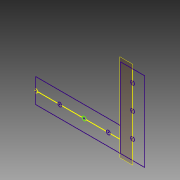
# Autodesk Inventor part: Bumper Holder
Saved by Autodesk Inventor 2014 (Build 180170000, 170)
## iProperties
Created: 2014-01-19
Part Number: Bumper Holder
Material: Generic
Document SubType Name: Sheet Metal
Designer: intern
Density: 1 g/cm^3
Sheet Metal Rule: Default
Appearance: Default
Author: intern
Autodesk Inventor part; units mm, degrees
ref_plane "YZ Plane" through (0, 0, 0) normal (1, 0, 0) x (0, 1, 0)
ref_plane "XZ Plane" through (0, 0, 0) normal (0, 1, 0) x (-1, 0, 0)
ref_plane "XY Plane" through (0, 0, 0) normal (0, 0, 1) x (1, 0, 0)
ref_plane "Work Plane1" through (7.5537, -38.3367, 0) normal (0, 0, 1) x (1, 0, 0)
sketch "Sketch1" plane through (7.5537, -38.3367, 0) normal (0, 0, 1) x (1, 0, 0)
  line L0 (-7.5537, -44.8483) -> (5.0701, -44.8483)
  line L1 (5.0701, -44.8483) -> (5.0701, -27.232)
  arc A0 (5.0701, -23.0946) -> (5.0701, -27.232) centre (5.1463, -25.1633) ccw
  line L2 (5.0701, -23.0946) -> (5.0701, -1.832)
  arc A1 (5.0701, 2.3054) -> (5.0701, -1.832) centre (5.1463, 0.2367) ccw
  line L3 (5.0701, 2.3054) -> (5.0701, 23.568)
  arc A2 (5.0701, 27.7054) -> (5.0701, 23.568) centre (5.1463, 25.6367) ccw
  line L4 (5.0701, 27.7054) -> (5.0701, 38.3367)
  line L5 (-7.5537, 38.3367) -> (5.0701, 38.3367)
  line L6 (-7.5537, 38.3367) -> (-7.5537, -44.8483)
  line L7 (5.2225, -44.8483) -> (17.8463, -44.8483)
  line L8 (17.8463, 38.3367) -> (17.8463, -44.8483)
  line L9 (5.2225, 38.3367) -> (17.8463, 38.3367)
  line L10 (5.2225, 27.7054) -> (5.2225, 38.3367)
  arc A3 (5.2225, 23.568) -> (5.2225, 27.7054) centre (5.1463, 25.6367) ccw
  line L11 (5.2225, 2.3054) -> (5.2225, 23.568)
  arc A4 (5.2225, -1.832) -> (5.2225, 2.3054) centre (5.1463, 0.2367) ccw
  line L12 (5.2225, -23.0946) -> (5.2225, -1.832)
  arc A5 (5.2225, -27.232) -> (5.2225, -23.0946) centre (5.1463, -25.1633) ccw
  line L13 (5.2225, -44.8483) -> (5.2225, -27.232)
  line L14 (-96.4537, -34.2184) -> (-96.4537, -44.8483)
  line L15 (-7.5537, -44.8483) -> (-96.4537, -44.8483)
  line L16 (-7.5537, -32.2245) -> (-7.5537, -44.8483)
  line L17 (-18.185, -32.2245) -> (-7.5537, -32.2245)
  arc A6 (-22.3224, -32.2245) -> (-18.185, -32.2245) centre (-20.2537, -32.1483) ccw
  line L18 (-43.585, -32.2245) -> (-22.3224, -32.2245)
  arc A7 (-47.7224, -32.2245) -> (-43.585, -32.2245) centre (-45.6537, -32.1483) ccw
  line L19 (-68.985, -32.2245) -> (-47.7224, -32.2245)
  arc A8 (-73.1224, -32.2245) -> (-68.985, -32.2245) centre (-71.0537, -32.1483) ccw
  line L20 (-94.385, -32.2245) -> (-73.1224, -32.2245)
  arc A9 (-96.4537, -34.2184) -> (-94.385, -32.2245) centre (-96.4537, -32.1483) ccw
  line L21 (-96.4537, -19.4483) -> (-96.4537, -30.0782)
  arc A10 (-94.385, -32.0721) -> (-96.4537, -30.0782) centre (-96.4537, -32.1483) ccw
  line L22 (-94.385, -32.0721) -> (-73.1224, -32.0721)
  arc A11 (-68.985, -32.0721) -> (-73.1224, -32.0721) centre (-71.0537, -32.1483) ccw
  line L23 (-68.985, -32.0721) -> (-47.7224, -32.0721)
  arc A12 (-43.585, -32.0721) -> (-47.7224, -32.0721) centre (-45.6537, -32.1483) ccw
  line L24 (-43.585, -32.0721) -> (-22.3224, -32.0721)
  arc A13 (-18.185, -32.0721) -> (-22.3224, -32.0721) centre (-20.2537, -32.1483) ccw
  line L25 (-18.185, -32.0721) -> (-7.5537, -32.0721)
  line L26 (-7.5537, -19.4483) -> (-7.5537, -32.0721)
  line L27 (-7.5537, -19.4483) -> (-96.4537, -19.4483)
  line L28 (-7.5537, 38.3367) -> (17.8463, 38.3367)
  line L29 (17.8463, 38.3367) -> (17.8463, -44.8483)
  line L30 (17.8463, -44.8483) -> (-7.5537, -44.8483)
  line L31 (-7.5537, -44.8483) -> (-7.5537, 38.3367)
  line L32 (-96.4537, -19.4483) -> (-7.5537, -19.4483)
  line L33 (-7.5537, -19.4483) -> (-7.5537, -44.8483)
  line L34 (-7.5537, -44.8483) -> (-96.4537, -44.8483)
  line L35 (-96.4537, -44.8483) -> (-96.4537, -19.4483)
  circle A14 centre (5.1463, -25.1633) radius 2.0701
  circle A15 centre (5.1463, 0.2367) radius 2.0701
  circle A16 centre (-45.6537, -32.1483) radius 2.0701
  circle A17 centre (-20.2537, -32.1483) radius 2.0701
  circle A18 centre (-71.0537, -32.1483) radius 2.0701
  circle A19 centre (5.1463, 25.6367) radius 2.0701
extrude "Plate1" add sketch "Sketch1" along normal blind 3.175 contours L6 L5 L4 A2 L3 A1 L2 A0 L1 L0 | L15 L14 A9 L20 A8 L19 A7 L18 A6 L17 L6 | L1 A14 L13 L30 | L17 A17 L25 L6 | L13 A5 L12 A4 L11 A3 L10 L9 L8 L7 | L25 A13 L24 A12 L23 A11 L22 A10 L21 L27 L6 | L35 A10 L22 A18 L20 A9 | L2 A15 L12 A14 | L18 A16 L24 A17 | L3 A19 L11 A15 | L10 A19 L4 L28 | L19 A18 L23 A16
fillet "Corner Round1" radius 6.35 6 edges at (0, 0, 1.5875) (25.4, 0, 1.5875) (-88.9, -57.785, 1.5875) (-88.9, -83.185, 1.5875) (0, -57.785, 1.5875) (25.4, -83.185, 1.5875)
equation "\"BendRadius\" = Thickness"
equation "\"BendReliefWidth\" = Thickness"
equation "\"BendReliefDepth\" = 0.5 * Thickness"
equation "\"CornerReliefSize\" = 4 * Thickness"
equation "\"MinimumRemnant\" = 2 * Thickness"
equation "\"TransitionRadius\" = BendRadius"
equation "\"JacobiRadiusSize\" = BendRadius"
equation "\"GapSize\" = Thickness"
equation "\"d0\" = BendRadius"
equation "\"Thickness\" = 3.175"
body "Solid1"
